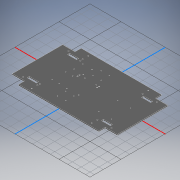
# Autodesk Inventor part: 000.001.002 - Днище
Saved by Autodesk Inventor 2022 (Build 260153000, 153)
## iProperties
Created: 2022-02-23
Part Number: 000.001.002 - Днище
Material: Типовые
Document SubType Name: Modeling
Designer: Petrov Ivan
Density: 1 g/cm^3
Appearance: По умолчанию(1)
Author: Petrov Ivan
Autodesk Inventor part; units mm, degrees
ref_plane "YZ Plane" through (0, 0, 0) normal (1, 0, 0) x (0, 1, 0)
ref_plane "XZ Plane" through (0, 0, 0) normal (0, 1, 0) x (-1, 0, 0)
ref_plane "XY Plane" through (0, 0, 0) normal (0, 0, 1) x (1, 0, 0)
sketch "Эскиз1" plane through (0, 0, 0) normal (0, 1, 0) x (-1, 0, 0)
  line L0 (-238, 142) -> (238, 142)
  line L1 (238, 142) -> (238, -142)
  line L2 (238, -142) -> (-238, -142)
  line L3 (-238, -142) -> (-238, 142)
  line L4 (-238, 142) -> (238, -142) construction
  line L5 (238, 142) -> (-238, -142) construction
  circle A0 centre (-139.231, 22.646) radius 2
  point P0 (0, 0)
  dimension "d0" = 476
  dimension "d1" = 284
  dimension "d10" = 4
  constraints: 12 end point, 2 midpoint, 2 parallel, 1 centre point, 1 horizontal, 1 perpendicular
  measures "d0" distance of L1.end L2.end
  measures "d1" distance of L0.end L1.end
  measures "d10" diameter of A0
extrude "Выдавливание1" add sketch "Эскиз1" along normal blind 4 contours L0 L1 L2 L3 | A0
sketch "Эскиз2" plane through (0, 4, 0) normal (0, 1, 0) x (1, 0, 0)
  line L0 (-238, -142) -> (238, -142) projected
  line L1 (-238, -142) -> (-182, -142)
  line L2 (-182, -142) -> (-182, -114)
  line L3 (-182, -114) -> (-238, -114)
  line L4 (-238, -114) -> (-238, -142)
  point P0 (0, 0)
  dimension "d4" = 56
  dimension "d5" = 28
  constraints: 8 end point, 2 parallel, 1 horizontal, 1 perpendicular
  measures "d4" distance of L3.end L2.end
  measures "d5" distance of L2.end L1.end
extrude "Выдавливание2" cut sketch "Эскиз2" against normal blind 4
mirror "Зеркальное отражение1" about plane through (0, 0, 0) normal (1, 0, 0) of "Выдавливание2"
mirror "Зеркальное отражение2" about plane through (0, 0, 0) normal (0, 0, 1) of "Выдавливание2", "Зеркальное отражение1"
sketch "Эскиз9" plane through (0, 0, 0) normal (0, -1, 0) x (1, 0, 0)
  circle A0 centre (-200, -128) radius 2.35 projected
  circle A1 centre (-136, -128) radius 2.35 projected
  circle A2 centre (-136, -128) radius 2.35 projected
  circle A3 centre (-136, -128) radius 2.35 projected
  circle A4 centre (-136, -102.6) radius 2.35 projected
  circle A5 centre (-200, -102.6) radius 2.35 projected
  circle A6 centre (-136, 102.6) radius 2.35 projected
  circle A7 centre (-136, 128) radius 2.35 projected
  circle A8 centre (-200, 102.6) radius 2.35 projected
  circle A9 centre (-200, 102.6) radius 2.35 projected
  circle A10 centre (-200, 102.6) radius 2.35 projected
  circle A11 centre (-200, 128) radius 2.35 projected
  circle A12 centre (200, 102.6) radius 2.35 projected
  circle A13 centre (200, 128) radius 2.35 projected
  circle A14 centre (136, 128) radius 2.35 projected
  circle A15 centre (136, 102.6) radius 2.35 projected
  circle A16 centre (200, -102.6) radius 2.35 projected
  circle A17 centre (200, -128) radius 2.35 projected
  circle A18 centre (136, -102.6) radius 2.35 projected
  circle A19 centre (136, -128) radius 2.35 projected
  point P0 (0, 0)
extrude "Выдавливание9" cut sketch "Эскиз9" against normal blind 10
sketch "Эскиз10" plane through (0, 0, 0) normal (0, -1, 0) x (1, 0, 0)
  line L0 (188.5, -86.25) -> (147.5, -86.25) projected
  line L1 (188.5, -96.25) -> (188.5, -86.25) projected
  line L2 (147.5, -96.25) -> (147.5, -86.25) projected
  line L3 (147.5, 96.25) -> (147.5, 86.25) projected
  line L4 (147.5, 86.25) -> (188.5, 86.25) projected
  line L5 (188.5, 96.25) -> (188.5, 86.25) projected
  line L6 (-188.5, 96.25) -> (-188.5, 86.25) projected
  line L7 (-188.5, 86.25) -> (-147.5, 86.25) projected
  line L8 (-147.5, 96.25) -> (-147.5, 86.25) projected
  line L9 (-188.5, -96.25) -> (-188.5, -86.25) projected
  line L10 (-147.5, -86.25) -> (-188.5, -86.25) projected
  line L11 (-147.5, -96.25) -> (-147.5, -86.25) projected
  line L12 (-188.5, 96.25) -> (-147.5, 96.25)
  line L13 (-147.5, 96.25) -> (-147.5, 86.25)
  line L14 (-147.5, 86.25) -> (-188.5, 86.25)
  line L15 (-188.5, 86.25) -> (-188.5, 96.25)
  line L16 (147.5, 96.25) -> (188.5, 96.25)
  line L17 (188.5, 96.25) -> (188.5, 86.25)
  line L18 (188.5, 86.25) -> (147.5, 86.25)
  line L19 (147.5, 86.25) -> (147.5, 96.25)
  line L20 (147.5, -96.25) -> (188.5, -96.25)
  line L21 (188.5, -96.25) -> (188.5, -86.25)
  line L22 (188.5, -86.25) -> (147.5, -86.25)
  line L23 (147.5, -86.25) -> (147.5, -96.25)
  line L24 (-188.5, -96.25) -> (-147.5, -96.25)
  line L25 (-147.5, -96.25) -> (-147.5, -86.25)
  line L26 (-147.5, -86.25) -> (-188.5, -86.25)
  line L27 (-188.5, -86.25) -> (-188.5, -96.25)
  point P0 (0, 0)
  constraints: 32 end point, 8 parallel, 4 horizontal, 4 perpendicular
extrude "Выдавливание10" cut sketch "Эскиз10" against normal blind 10
sketch "Эскиз11" plane through (0, 0, 0) normal (0, -1, 0) x (1, 0, 0)
  circle A0 centre (165, -18.75) radius 1.375 projected
  circle A1 centre (107, -18.75) radius 1.375 projected
  circle A2 centre (107, 67.25) radius 1.375 projected
  circle A3 centre (165, 67.25) radius 1.375 projected
  circle A4 centre (-11.1434, -98.825) radius 1.5 projected
  circle A5 centre (-48.1434, -98.825) radius 1.5 projected
  circle A6 centre (-11.1434, -61.825) radius 1.5 projected
  circle A7 centre (-48.1434, -61.825) radius 1.5 projected
  circle A8 centre (-4.2432, -32.6475) radius 1.75 projected
  circle A9 centre (-56.3132, -32.6475) radius 1.75 projected
  circle A10 centre (-56.3132, 48.6325) radius 1.75 projected
  circle A11 centre (-4.2432, 47.3625) radius 1.75 projected
  circle A12 centre (-11.1434, 61.825) radius 1.5 projected
  circle A13 centre (-11.1434, 98.825) radius 1.5 projected
  circle A14 centre (-48.1434, 98.825) radius 1.5 projected
  circle A15 centre (-48.1434, 61.825) radius 1.5 projected
  circle A16 centre (-124.63, 46.96) radius 1.6 projected
  circle A17 centre (-92.88, 46.96) radius 1.6 projected
  circle A18 centre (-92.88, -14) radius 1.6 projected
  circle A19 centre (-124.63, -14) radius 1.6 projected
  circle A20 centre (-74.28, -83.71) radius 1.75 projected
  circle A21 centre (-116.19, -83.71) radius 1.75 projected
  circle A22 centre (-74.28, -44.34) radius 1.75 projected
  circle A23 centre (-116.19, -44.34) radius 1.75 projected
  line L0 (-78.15, -33.46) -> (-78.15, -32.16) projected
  line L1 (-78.15, -32.16) -> (-79.6, -30.71) projected
  line L2 (-79.6, -30.71) -> (-80.9, -30.71) projected
  line L3 (-80.9, -30.71) -> (-82.35, -32.16) projected
  line L4 (-82.35, -32.16) -> (-82.35, -33.46) projected
  line L5 (-82.35, -33.46) -> (-80.9, -34.91) projected
  line L6 (-80.9, -34.91) -> (-79.6, -34.91) projected
  line L7 (-79.6, -34.91) -> (-78.15, -33.46) projected
  line L8 (-81.65, -33.1701) -> (-80.6101, -34.21) projected
  line L9 (-81.65, -32.4499) -> (-81.65, -33.1701) projected
  line L10 (-80.6101, -31.41) -> (-81.65, -32.4499) projected
  line L11 (-79.8899, -31.41) -> (-80.6101, -31.41) projected
  line L12 (-78.85, -32.4499) -> (-79.8899, -31.41) projected
  line L13 (-78.85, -33.1701) -> (-78.85, -32.4499) projected
  line L14 (-79.8899, -34.21) -> (-78.85, -33.1701) projected
  line L15 (-80.6101, -34.21) -> (-79.8899, -34.21) projected
  line L16 (-78.15, -24.46) -> (-78.15, -23.16) projected
  line L17 (-78.15, -23.16) -> (-79.6, -21.71) projected
  line L18 (-79.6, -21.71) -> (-80.9, -21.71) projected
  line L19 (-80.9, -21.71) -> (-82.35, -23.16) projected
  line L20 (-82.35, -23.16) -> (-82.35, -24.46) projected
  line L21 (-82.35, -24.46) -> (-80.9, -25.91) projected
  line L22 (-80.9, -25.91) -> (-79.6, -25.91) projected
  line L23 (-79.6, -25.91) -> (-78.15, -24.46) projected
  line L24 (-81.65, -24.1701) -> (-80.6101, -25.21) projected
  line L25 (-81.65, -23.4499) -> (-81.65, -24.1701) projected
  line L26 (-80.6101, -22.41) -> (-81.65, -23.4499) projected
  line L27 (-79.8899, -22.41) -> (-80.6101, -22.41) projected
  line L28 (-78.85, -23.4499) -> (-79.8899, -22.41) projected
  line L29 (-78.85, -24.1701) -> (-78.85, -23.4499) projected
  line L30 (-79.8899, -25.21) -> (-78.85, -24.1701) projected
  line L31 (-80.6101, -25.21) -> (-79.8899, -25.21) projected
  line L32 (10.75, -24.46) -> (10.75, -23.16) projected
  line L33 (10.75, -23.16) -> (9.3, -21.71) projected
  line L34 (9.3, -21.71) -> (8, -21.71) projected
  line L35 (8, -21.71) -> (6.55, -23.16) projected
  line L36 (6.55, -23.16) -> (6.55, -24.46) projected
  line L37 (6.55, -24.46) -> (8, -25.91) projected
  line L38 (8, -25.91) -> (9.3, -25.91) projected
  line L39 (9.3, -25.91) -> (10.75, -24.46) projected
  line L40 (7.25, -24.1701) -> (8.2899, -25.21) projected
  line L41 (7.25, -23.4499) -> (7.25, -24.1701) projected
  line L42 (8.2899, -22.41) -> (7.25, -23.4499) projected
  line L43 (9.0101, -22.41) -> (8.2899, -22.41) projected
  line L44 (10.05, -23.4499) -> (9.0101, -22.41) projected
  line L45 (10.05, -24.1701) -> (10.05, -23.4499) projected
  line L46 (9.0101, -25.21) -> (10.05, -24.1701) projected
  line L47 (8.2899, -25.21) -> (9.0101, -25.21) projected
  line L48 (10.75, -33.46) -> (10.75, -32.16) projected
  line L49 (10.75, -32.16) -> (9.3, -30.71) projected
  line L50 (9.3, -30.71) -> (8, -30.71) projected
  line L51 (8, -30.71) -> (6.55, -32.16) projected
  line L52 (6.55, -32.16) -> (6.55, -33.46) projected
  line L53 (6.55, -33.46) -> (8, -34.91) projected
  line L54 (8, -34.91) -> (9.3, -34.91) projected
  line L55 (9.3, -34.91) -> (10.75, -33.46) projected
  line L56 (7.25, -33.1701) -> (8.2899, -34.21) projected
  line L57 (7.25, -32.4499) -> (7.25, -33.1701) projected
  line L58 (8.2899, -31.41) -> (7.25, -32.4499) projected
  line L59 (9.0101, -31.41) -> (8.2899, -31.41) projected
  line L60 (10.05, -32.4499) -> (9.0101, -31.41) projected
  line L61 (10.05, -33.1701) -> (10.05, -32.4499) projected
  line L62 (9.0101, -34.21) -> (10.05, -33.1701) projected
  line L63 (8.2899, -34.21) -> (9.0101, -34.21) projected
  circle A24 centre (-135.5, -91.25) radius 2.775 projected
  circle A25 centre (-135.5, 91.25) radius 2.775 projected
  point P0 (0, 0)
extrude "Выдавливание11" cut sketch "Эскиз11" against normal blind 10 contours A0 | A1 | A2 | A3 | A4 | A5 | A6 | A7 | A8 | A9 | A10 | A11 | A12 | A13 | A14 | A15 | A16 | A17 | A18 | A19 | A20 | A21 | A22 | A23 | L7 L6 L5 L4 L3 L2 L1 L0 | L9 L10 L11 L12 L13 L14 L15 L8 | L23 L22 L21 L20 L19 L18 L17 L16 | L25 L26 L27 L28 L29 L30 L31 L24 | L39 L38 L37 L36 L35 L34 L33 L32 | L41 L42 L43 L44 L45 L46 L47 L40 | L55 L54 L53 L52 L51 L50 L49 L48 | L57 L58 L59 L60 L61 L62 L63 L56 | A24 | A25
